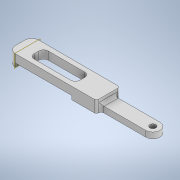
# Autodesk Inventor part: SideSensor_Mount
Saved by Autodesk Inventor 2022 (Build 260153000, 153)
## iProperties
Created: 2022-09-16
Part Number: SideSensor_Mount
Material: 一般
Document SubType Name: Modeling
Designer: Yazawa
Density: 1 g/cm^3
Appearance: 既定
Author: Yazawa
Autodesk Inventor part; units mm, degrees
ref_plane "YZ Plane" through (0, 0, 0) normal (1, 0, 0) x (0, 1, 0)
ref_plane "XZ Plane" through (0, 0, 0) normal (0, 1, 0) x (-1, 0, 0)
ref_plane "XY Plane" through (0, 0, 0) normal (0, 0, 1) x (1, 0, 0)
sketch "スケッチ1" plane through (0, 0, 0) normal (0, 1, 0) x (-1, 0, 0)
  line L0 (37.5, -5) -> (0, -5)
  line L1 (0, -5) -> (0, 5)
  line L2 (0, 5) -> (37.5, 5)
  line L3 (37.5, 5) -> (37.5, -5)
  line L4 (0, -3) -> (-22, -3)
  line L5 (-22, -3) -> (-22, 3)
  line L6 (-22, 3) -> (0, 3)
  line L7 (0, 3) -> (0, -3)
  line L8 (0, 0) -> (-22, 0) construction
  line L9 (0, 0) -> (37.5, 0) construction
  point P0 (0, 3)
  dimension "d1" = 22
  dimension "d2" = 10
  dimension "d3" = 6
  dimension "d17" = 59.5
  constraints: 20 end point, 5 midpoint, 4 parallel, 2 horizontal, 2 perpendicular, 1 coincident, 1 collinear, 1 point on line
  measures "d1" distance of L4.start L4.end
  measures "d2" distance of L2.end L0.start
  measures "d3" distance between parallel lines of L4 L6
  measures "d17" distance between parallel lines of L5 L3
extrude "押し出し1" add sketch "スケッチ1" along normal blind 5
sketch "スケッチ2" plane through (0, 5, 0) normal (0, 1, 0) x (1, 0, 0)
  line L0 (22, 3) -> (0, 3) projected
  line L1 (0, 5) -> (-37.5, 5) projected
  line L2 (-37.5, 5) -> (-37.5, -5) projected
  line L3 (-37.5, -5) -> (0, -5) projected
  line L4 (0, -3) -> (22, -3) projected
  line L5 (0, 3) -> (0, 5) projected
  line L6 (0, -5) -> (0, -3) projected
  line L7 (22, -3) -> (22, 3) projected
  line L8 (0, 3) -> (0, -3)
  point P0 (0, 0)
  constraints: 2 end point, 1 vertical
extrude "押し出し3" cut sketch "スケッチ2" against normal blind 2.5 contours L7 L4 L8 L0
ref_plane "作業平面2" through (-34.5, 0, -5) normal (-1, 0, 0) x (0, 0, 1)
fillet "フィレット5" radius 3 4 edges at (22, 1.25, 3) (22, 1.25, -3) (-37.5, 2.5, 5) (-37.5, 2.5, -5)
fillet "フィレット6" radius 1 4 edges at (0, 2.5, 5) (0, 2.5, -5) (0, 1.25, 3) (0, 1.25, -3)
fillet "フィレット7" radius 1.25 3 edges at (0, 2.5, 3.4999) (0, 2.5, 0) (0, 2.5, -3.5)
sketch "スケッチ5" plane through (0, 0, 0) normal (0, -1, 0) x (1, 0, 0)
  arc A0 (19, -3) -> (19, 3) centre (19, 0) ccw projected
  point P0 (0, 0)
hole "穴1" at (19, 0, 0) direction (0, 1, 0) diameter 2.5 end through all
sketch "スケッチ6" plane through (0, 0, 0) normal (0, -1, 0) x (1, 0, 0)
  line L0 (-34.5, 5) -> (-34.5, 0)
  line L1 (-6.5, 0) -> (-6.5, 3)
  line L2 (-6.5, 3) -> (-10.5, 3)
  line L3 (-10.5, 3) -> (-10.5, 5)
  line L4 (-34.5, 0) -> (-6.5, 0) construction
  line L5 (-34.5, 5) -> (-10.5, 5)
  line L6 (-37.5, -2) -> (-37.5, 2) projected
  line L7 (-34.5, -5) -> (-34.5, 0)
  line L8 (-6.5, 0) -> (-6.5, -3)
  line L9 (-6.5, -3) -> (-10.5, -3)
  line L10 (-10.5, -3) -> (-10.5, -5)
  line L11 (-34.5, -5) -> (-10.5, -5)
  point P0 (0, 0)
  dimension "d31" = 3
  dimension "d32" = 28
  dimension "d33" = 4
  dimension "d35" = 10
  dimension "d36" = 6
  constraints: 22 end point, 4 symmetric about line, 3 perpendicular, 2 horizontal, 1 point on line, 1 vertical
  measures "d31" distance between parallel lines of L6 L0
  measures "d32" distance between parallel lines of L1 L0
  measures "d33" distance of L1.end L2.end
  measures "d35" distance between parallel lines of L11 L5
  measures "d36" distance between parallel lines of L9 L2
extrude "押し出し4" cut sketch "スケッチ6" against normal blind 1.6
sketch "スケッチ7" plane through (0, 1.6, 0) normal (0, -1, 0) x (1, 0, 0)
  line L0 (-10.5, 3) -> (-6.5, 3) projected
  line L1 (-10.5, 5) -> (-10.5, 3) projected
  line L2 (-34.5, 5) -> (-10.5, 5) projected
  line L3 (-34.5, -5) -> (-34.5, 5) projected
  line L4 (-10.5, -5) -> (-34.5, -5) projected
  line L5 (-10.5, -3) -> (-10.5, -5) projected
  line L6 (-6.5, -3) -> (-10.5, -3) projected
  line L7 (-6.5, 3) -> (-6.5, -3) projected
  line L8 (-6.5, 3) -> (-6.5, -3) construction
  line L9 (-6.5, 0) -> (-34.5, 0) construction
  point P0 (0, 0)
  point P1 (-8.5, 0)
  point P2 (-32.5, 0)
  dimension "d39" = 2
  dimension "d40" = 2
  constraints: 2 end point, 2 midpoint, 2 point on line
  measures "d39" distance from line of L3 point (-32.5, 0)
  measures "d40" distance from line of L7 point (-8.5, 0)
hole "穴2" at (-8.5, 1.6, 0) at (-32.5, 1.6, 0) direction (0, 1, 0) diameter 1 depth 0.1 tip angle 118
sketch "スケッチ8" plane through (0, 1.6, 0) normal (0, -1, 0) x (1, 0, 0)
  line L0 (-13, 3) -> (-28.5, 3)
  line L1 (-30.5, 1) -> (-30.5, -1)
  line L2 (-28.5, -3) -> (-13, -3)
  line L3 (-11, -1) -> (-11, 1)
  line L4 (-11, 0) -> (-30.5, 0) construction
  line L5 (-6.5, 3) -> (-6.5, -3) construction
  circle A0 centre (-8.5, 0) radius 0.5 projected
  circle A1 centre (-32.5, 0) radius 0.5 projected
  arc A2 (-11, 1) -> (-13, 3) centre (-13, 1) ccw
  arc A3 (-13, -3) -> (-11, -1) centre (-13, -1) ccw
  arc A4 (-30.5, -1) -> (-28.5, -3) centre (-28.5, -1) ccw
  arc A5 (-28.5, 3) -> (-30.5, 1) centre (-28.5, 1) ccw
  point P0 (0, 0)
  point P1 (-11, 3)
  point P2 (-11, -3)
  dimension "d48" = 19.5
  dimension "d49" = 6
  dimension "d50" = 2.5
  dimension "d51" = 2
  constraints: 10 end point, 8 point on circle, 8 tangent, 5 point on line, 4 centre point, 3 equal radius, 2 midpoint, 2 parallel, 1 horizontal, 1 perpendicular
  measures "d48" distance between parallel lines of L1 L3
  measures "d49" distance of point (-11, -3) point (-11, 3)
  measures "d50" distance from line of A0.centre L3
  measures "d51" radius of A2
extrude "押し出し5" cut sketch "スケッチ8" against normal through all contours A2 L3 A3 L2 A4 L1 A5 L0
